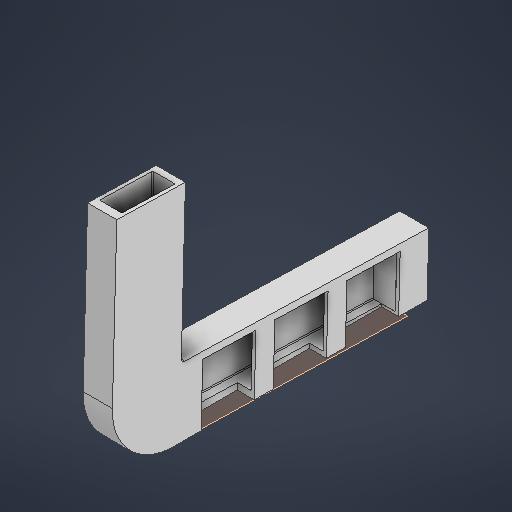
# Autodesk Inventor part: CoinFeeder
Saved by Autodesk Inventor 2026.3 (Build 303398000, 398)
## iProperties
Created: 2026-05-04
Part Number: CoinFeeder
Material: Generic
Document SubType Name: Modeling
Designer: frede
Density: 1 g/cm^3
Appearance: Default
Author: frede
Autodesk Inventor part; units mm, degrees
ref_plane "YZ Plane" through (0, 0, 0) normal (1, 0, 0) x (0, 1, 0)
ref_plane "XZ Plane" through (0, 0, 0) normal (0, 1, 0) x (-1, 0, 0)
ref_plane "XY Plane" through (0, 0, 0) normal (0, 0, 1) x (1, 0, 0)
sketch "Sketch2" plane through (0, 0, 0) normal (1, 0, 0) x (0, 1, 0)
  line L0 (0, 148.2335) -> (4.9982, 148.0987)
  line L1 (4.9982, 148.0987) -> (1.0018, -0.027)
  line L2 (1.0018, -0.027) -> (31.9905, -0.8631)
  line L3 (35.8251, 141.2648) -> (31.9905, -0.8631)
  line L4 (31.9905, -0.8631) -> (35.9891, -0.971)
  arc A0 (36.9578, 183.2495) -> (0, 148.2335) centre (35.9869, 147.2626) ccw
  line L5 (41.9847, 147.1008) -> (129.9527, 144.7275)
  line L6 (36.9578, 183.2495) -> (130.9236, 180.7144)
  arc A1 (36.823, 178.2513) -> (4.9982, 148.0987) centre (35.9869, 147.2626) ccw
  line L7 (36.823, 178.2513) -> (130.7888, 175.7162)
  line L8 (130.9236, 180.7144) -> (130.7888, 175.7162)
  line L9 (129.8448, 140.7289) -> (41.8768, 143.1022)
  line L10 (39.9855, 147.1548) -> (39.9855, 147.1547)
  line L11 (39.8236, 141.1569) -> (35.9891, -0.971)
  arc A2 (41.8768, 143.1022) -> (39.8236, 141.1569) centre (41.8229, 141.103) ccw
  line L12 (0, 148.2335) -> (0, 0)
  line L13 (129.9527, 144.7275) -> (129.8448, 140.7289)
  line L14 (1.0018, -0.027) -> (0, 0)
  arc A3 (41.9847, 147.1008) -> (35.8251, 141.2648) centre (41.8229, 141.103) ccw
  line L15 (0, 16.5) -> (36.4339, 15.517)
  line L16 (130.7888, 175.7162) -> (129.9527, 144.7275)
  point P0 (65.823, 177.4689)
  point P1 (32.4354, 15.6249)
  point P2 (1.4467, 16.461)
  dimension "d1" = 5
  dimension "d10" = 2
  dimension "d11" = 6
  dimension "d12" = 31
  dimension "d13" = 5
  dimension "d14" = 31
  dimension "d15" = 4
  dimension "d17" = 4
  dimension "d42" = 90
  constraints: 34 end point, 8 point on circle, 7 perpendicular, 6 parallel, 4 centre point, 4 tangent, 3 point on line, 1 coincident, 1 vertical
  measures "d1" distance of L0.start L0.end
  measures "d10" radius of A2
  measures "d11" radius of A3
  measures "d12" distance between parallel lines of L1 L3
  measures "d13" distance between parallel lines of L7 L6
  measures "d14" distance between parallel lines of L5 L7
  measures "d15" distance between parallel lines of L9 L5
  measures "d17" distance between parallel lines of L3 L11
  measures "d42" distance between parallel lines of L11 L8
extrude "Extrusion1" add sketch "Sketch2" against normal blind 2
extrude "Extrusion2" add sketch "Sketch2" along normal blind 13 contours A0 L6 L8 L7 A1 L0 | L0 L1 L15 L12 | L15 L1 L14 L12 | L15 L3 L2 L1 | L15 L11 L4 L3 | L3 A3 L5 L13 L9 A2 L11 L15
sketch "Sketch4" plane through (13, 0, 0) normal (1, 0, 0) x (0, 0, -1)
  line L0 (-180.7144, 130.9236) -> (-183.2495, 36.9578) projected
  arc A0 (-183.2495, 36.9578) -> (-148.2335, 0) centre (-147.2626, 35.9869) ccw projected
  line L1 (-148.2335, 0) -> (0, 0) projected
  line L2 (0, 0) -> (0.027, 1.0018) projected
  line L3 (0.027, 1.0018) -> (0.8631, 31.9905) projected
  line L4 (0.8631, 31.9905) -> (0.971, 35.9891) projected
  line L5 (0.971, 35.9891) -> (-141.1569, 39.8236) projected
  arc A1 (-143.1022, 41.8768) -> (-141.1569, 39.8236) centre (-141.103, 41.8229) ccw projected
  line L6 (-143.1022, 41.8768) -> (-140.7289, 129.8448) projected
  line L7 (-140.7289, 129.8448) -> (-144.7275, 129.9527) projected
  line L8 (-146.4802, 64.9869) -> (-177.4689, 65.823) projected
  line L9 (-144.7275, 129.9527) -> (-180.7144, 130.9236) projected
  point P0 (-177.4689, 65.823)
  constraints: 1 other
extrude "Extrusion3" add sketch "Sketch4" along normal blind 2
ref_plane "Work Plane1" through (0, 0, 148.2335) normal (0, 0.9996363, -0.0269697) x (1, 0, 0)
sketch "Sketch8" plane through (0, 0, 148.2335) normal (0, 0.9996363, -0.0269697) x (1, 0, 0)
  line L0 (0, 0) -> (0, 131.6856) projected
  line L1 (0, 0) -> (13, 0) projected
  line L2 (13, 131.6856) -> (13, 0) projected
  line L3 (0, 131.6856) -> (13, 131.6856) projected
  line L4 (15, 148.1796) -> (-2, 148.1796) projected
  line L5 (15, 58.5898) -> (5, 58.5898)
  line L6 (5, 58.5898) -> (5, 89.5898)
  line L7 (5, 89.5898) -> (15, 89.5898)
  line L8 (15, 89.5898) -> (15, 58.5898)
  line L9 (15, 16.5898) -> (5, 16.5898)
  line L10 (5, 16.5898) -> (5, 47.5898)
  line L11 (5, 47.5898) -> (15, 47.5898)
  line L12 (15, 47.5898) -> (15, 16.5898)
  line L13 (15, 100.5898) -> (5, 100.5898)
  line L14 (5, 100.5898) -> (5, 131.5898)
  line L15 (5, 131.5898) -> (15, 131.5898)
  line L16 (15, 131.5898) -> (15, 100.5898)
  point P0 (0, 148.1796)
  point P1 (6.5, 74.0898)
  point P2 (6.5, 32.0898)
  point P3 (6.5, 116.0898)
  dimension "d45" = 148.1796
  dimension "d46" = 74.0898
  dimension "d47" = 10
  dimension "d48" = 31
  dimension "d49" = 15.5
  dimension "d50" = 10
  dimension "d53" = 42
  constraints: 24 end point, 2 parallel, 1 horizontal, 1 perpendicular, 1 vertical, 18 other
  measures "d45" distance between parallel lines of L1 L4
  measures "d46" distance from line of point (6.5, 74.09) L1
  measures "d47" distance of L6.end L7.end
  measures "d48" distance of L5.end L6.end
  measures "d49" distance from line of L5 point (6.5, 74.09)
  measures "d50" distance between parallel lines of L8 L6
  measures "d53" distance of L5.start L9.start
fillet "Fillet1" radius 0.5 12 edges at (0, 14.6658, 169.7661) (0, 83.8059, 176.9838) (0, 3.2224, 82.2798) (0, 37.6962, 145.4585) (0, 34.1302, 78.4449) (0, 85.9687, 145.9141) (13, 37.6962, 145.4585) (13, 34.1302, 78.4449) (13, 85.9687, 145.9141) (13, 14.6658, 169.7661) (13, 3.2224, 82.2798) (13, 83.8059, 176.9838)
extrude "Extrusion6" cut sketch "Sketch8" along normal blind 36 contours L9 L10 L11 L2 | L2 L11 L12 L9 | L15 L16 L13 L2 | L2 L13 L14 L15 | L5 L6 L7 L2 | L2 L7 L8 L5
equation "\"d46\" = 0.5 * d45"
equation "\"d49\" = 0.5 * d48"
body "Solid1"
